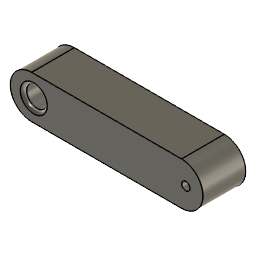
seminaire_FISA-A3_tige-servomotor_47mm (Autodesk Fusion 360 design; units mm, degrees)
part number: 2026-07-28-15-01-46-336
Autodesk Fusion 360 part; units mm, degrees
sketch "Esquisse1" plane through (0, 0, 0) normal (0, 0, 1) x (1, 0, 0)
  line L0 (-30, 25) -> (15, 25)
  line L1 (15, 25) -> (15, 15)
  line L2 (15, 15) -> (-30, 15)
  line L3 (-30, 15) -> (-30, 25)
  dimension "d21" = 10
  dimension "d22" = 45
  constraint horizontal L0
  constraint vertical L1
  constraint horizontal L2
  constraint vertical L3
  measures "d21" distance of L0.start L2.end
  measures "d22" distance of L1.end L2.end
extrude "Extrusion1" add sketch "Esquisse1" along normal blind 10
sketch "Esquisse2" plane through (0, 0, 0) normal (0, 1, 0) x (1, 0, 0)
  circle A0 centre (-24.5, -5) radius 2.4
  circle A1 centre (11, -5) radius 0.975
  line L0 (15, 0) -> (15, -10)
  line L1 (-30, 0) -> (-30, -10)
  dimension "d3" = 4.8
  dimension "d4" = 1.95
  dimension "d25" = 4
  dimension "d26" = 5.5
  measures "d3" diameter of A0
  measures "d4" diameter of A1
  measures "d25" distance of A1.centre L0
  measures "d26" distance of A0.centre L1
extrude "Extrusion2" cut sketch "Esquisse2" along normal blind 25 and the other way blind -15
fillet "Congé4" radius 5 4 edges at (-30, 20, 10) (15, 20, 10) (15, 20, 0) (-30, 20, 0)
fillet "Congé5" radius 0.75 2 edges at (-26.7376, 15, 5.8679) (-26.7376, 25, 4.1321)
